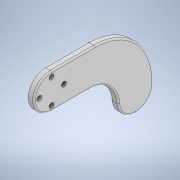
# Autodesk Inventor part: base9
Saved by Autodesk Inventor 2022 (Build 260153000, 153)
## iProperties
Created: 2022-06-16
Part Number: base9
Material: 一般
Document SubType Name: Modeling
Designer: yuto6
Density: 1 g/cm^3
Appearance: 既定
Author: yuto6
Autodesk Inventor part; units mm, degrees
ref_plane "YZ Plane" through (0, 0, 0) normal (1, 0, 0) x (0, 1, 0)
ref_plane "XZ Plane" through (0, 0, 0) normal (0, 1, 0) x (-1, 0, 0)
ref_plane "XY Plane" through (0, 0, 0) normal (0, 0, 1) x (1, 0, 0)
sketch "スケッチ1" plane through (0, 0, 0) normal (1, 0, 0) x (0, 1, 0)
  circle A0 centre (0, 0) radius 12
  line L0 (12, 0) -> (-12, 0)
  line L1 (-12, 0) -> (-12, -70)
  line L2 (-12, -70) -> (12, -70)
  line L3 (12, -70) -> (12, 0)
  line L4 (-12, -70) -> (-42, -70)
  line L5 (-42, -70) -> (-42, -46)
  line L6 (-42, -46) -> (-12, -46)
  line L7 (-12, -46) -> (-12, -70)
  point P0 (-12, -46)
  dimension "d0" = 24
  dimension "d1" = 70
  dimension "d4" = 24
  dimension "d5" = 30
  constraints: 16 end point, 4 parallel, 2 horizontal, 2 perpendicular, 2 vertical, 1 coincident, 3 other
  measures "d1" distance from line of point (0, 0) L2
  measures "d4" distance of L4.end L5.end
  measures "d5" distance between parallel lines of L1 L5
extrude "押し出し1" add sketch "スケッチ1" along normal blind 5
fillet "フィレット1" radius 20 1 edges at (2.5, -12, -46)
fillet "フィレット3" radius 40 1 edges at (2.5, 12, -70)
fillet "フィレット2" radius 12 2 edges at (2.5, -42, -46) (2.5, -42, -70)
sketch "スケッチ2" plane through (5, 0, 0) normal (1, 0, 0) x (0, 0, -1)
  circle A0 centre (0, 0) radius 8.5
  point P0 (0, 8.5)
  dimension "d8" = 17
  constraints: 1 coincident, 1 vertical alignment, 2 other
hole "穴1" at (5, 8.5, 0) direction (-1, 0, 0) diameter 3.4 end through all clearance for "Flat Head Machine Screw" size "M3" standard "Ansi Metric M Profile"
pattern_circular "円形状パターン1" count 4 over 360 about axis through (0, 0, 0) along (1, 0, 0) of "穴1"
fillet "フィレット4" radius 1 16 edges at (5, -29, -70) (5, -38.4853, -66.4853) (5, -42, -57.9687) (5, -38.7464, -49.7216) (5, -12, -13) (5, 0, 12) (5, 12, -15) (5, 0.2843, -58.2843) (0, 12, -15) (0, 0, 12) (0, -12, -13) (0, -38.7464, -49.7216) (0, -42, -57.9687) (0, -38.4853, -66.4853) (0, -29, -70) (0, 0.2843, -58.2843)
